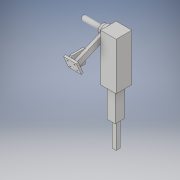
# Autodesk Inventor part: simp_burnisher
Saved by Autodesk Inventor 2019 (Build 230136000, 136)
## iProperties
Created: 2019-11-07
Part Number: simp_burnisher
Material: Generic
Document SubType Name: Modeling
Designer: luua
Density: 1 g/cm^3
Appearance: Default
Author: luua
Autodesk Inventor part; units mm, degrees
ref_plane "YZ Plane" through (0, 0, 0) normal (1, 0, 0) x (0, 1, 0)
ref_plane "XZ Plane" through (0, 0, 0) normal (0, 1, 0) x (-1, 0, 0)
ref_plane "XY Plane" through (0, 0, 0) normal (0, 0, 1) x (1, 0, 0)
sketch "Sketch1" plane through (0, 0, 0) normal (0, 0, 1) x (1, 0, 0)
  line L0 (-76.6085, 0) -> (76.6085, 0) construction
  line L1 (-48, 0) -> (48, 0)
  line L2 (48, 0) -> (48, 11)
  line L3 (48, 11) -> (-48, 11)
  line L4 (-48, 11) -> (-48, 0)
  point P0 (0, 0)
  point P1 (0, 0)
  point P2 (0, 11)
  dimension "d0" = 96
  dimension "d1" = 11
  constraints: 10 end point, 2 horizontal, 2 midpoint, 2 parallel, 1 coincident, 1 perpendicular, 1 point on line, 1 vertical alignment
  measures "d0" distance of L2.end L3.end
  measures "d1" distance of L1.end L2.end
revolve "Revolution1" add sketch "Sketch1" angle 360 about axis through (-76.6085, 0, 0) along (1, 0, 0)
sketch "Sketch2" plane through (48, 0, 0) normal (1, 0, 0) x (0, 0, -1)
  circle A0 centre (0, 0) radius 22.5
  dimension "d3" = 45
  constraints: 1 centre point, 1 coincident
  measures "d3" diameter of A0
extrude "Extrusion1" add sketch "Sketch2" along normal blind 30
sketch "Sketch3" plane through (0, 0, 0) normal (0, 0, 1) x (1, 0, 0)
  line L0 (78, -22.5) -> (78, 22.5) projected
  line L1 (78, 27.5) -> (78, -212.5)
  line L2 (48, 22.5) -> (78, 22.5) projected
  line L3 (48, -22.5) -> (78, -22.5) projected
  line L4 (78, 27.5) -> (158, 27.5)
  line L5 (158, 27.5) -> (158, -212.5)
  line L6 (78, -212.5) -> (98, -212.5)
  line L7 (158, -212.5) -> (138, -212.5)
  line L8 (118, 27.5) -> (118, -212.5) construction
  line L9 (98, -212.5) -> (98, -362.5)
  line L10 (98, -362.5) -> (138, -362.5)
  line L11 (138, -362.5) -> (138, -212.5)
  line L12 (108, -362.5) -> (128, -362.5)
  line L13 (128, -362.5) -> (128, -492.5)
  line L14 (128, -492.5) -> (108, -492.5)
  line L15 (108, -492.5) -> (108, -362.5)
  line L16 (138, -212.5) -> (98, -212.5)
  point P0 (0, 0)
  point P1 (118, -362.5)
  dimension "d6" = 5
  dimension "d7" = 190
  dimension "d8" = 80
  dimension "d9" = 40
  dimension "d10" = 150
  dimension "d36" = 20
  dimension "d37" = 130
  constraints: 28 end point, 6 horizontal, 3 midpoint, 3 perpendicular, 3 vertical, 2 collinear, 2 parallel, 1 horizontal alignment, 1 symmetric about line
  measures "d6" distance from line of L1.start L2
  measures "d7" distance from line of L1.end L3
  measures "d8" distance of L1.start L4.end
  measures "d9" distance of L6.end L7.end
  measures "d10" distance of L6.end L9.end
  measures "d36" distance of L13.end L14.end
  measures "d37" distance of L12.end L13.end
extrude "Extrusion2" add sketch "Sketch3" along normal mid plane 80 contours L0 L1 L4 L5 L7 L16 L6
sketch "Sketch4" plane through (78, -212.5, 40) normal (-1, 0, 0) x (0, 0, 1)
  circle A0 centre (-40, 212.5) radius 22.5 projected
  circle A1 centre (-40, 212.5) radius 27.5
  line L0 (-12.6869, 215.7005) -> (123.729, 157.7954)
  line L1 (123.729, 157.7954) -> (112.0071, 130.1803)
  line L2 (112.0071, 130.1803) -> (-26.0686, 188.7899)
  line L3 (0, 240) -> (0, 0) projected
  dimension "d13" = 55
  dimension "d14" = 150
  dimension "d15" = 90
  dimension "d16" = 30
  dimension "d17" = 67
  constraints: 6 end point, 2 point on circle, 1 centre point, 1 coincident, 1 perpendicular
  measures "d13" diameter of A1
  measures "d14" distance of L1.end L2.end
  measures "d15" angle of L1 L2
  measures "d16" distance of L0.end L1.end
  measures "d17" angle of L3 L2
extrude "Extrusion3" add sketch "Sketch4" along normal blind 15
extrude "Extrusion7" add sketch "Sketch3" along normal mid plane 50 contours L16 L11 L10 L9
extrude "Extrusion8" add sketch "Sketch3" along normal mid plane 20 contours L10 L13 L14 L15
sketch "Sketch5" plane through (63, -212.5, 40) normal (-1, 0, 0) x (0, 0, 1)
  line L0 (62.2205, 183.9042) -> (130.5668, 183.9042)
  line L1 (105.1693, 114.0714) -> (62.2205, 114.0714)
  line L2 (62.2205, 114.0714) -> (62.2205, 183.9042)
  line L3 (123.729, 157.7954) -> (-12.6869, 215.7005) projected
  circle A0 centre (-40, 212.5) radius 22.5 projected
  arc A1 (-12.6869, 215.7005) -> (-26.0686, 188.7899) centre (-40, 212.5) ccw projected
  line L4 (-26.0686, 188.7899) -> (112.0071, 130.1803) projected
  line L5 (112.0071, 130.1803) -> (123.729, 157.7954) projected
  line L6 (123.729, 157.7954) -> (-12.6869, 215.7005) projected
  line L7 (130.5668, 173.9042) -> (105.1693, 114.0714)
  line L8 (105.1693, 114.0714) -> (114.3743, 110.1641)
  line L9 (114.3743, 110.1641) -> (139.7719, 169.9969)
  line L10 (139.7719, 169.9969) -> (130.5668, 173.9042)
  line L11 (112.0071, 130.1803) -> (123.729, 157.7954) projected
  line L12 (130.5668, 183.9042) -> (130.5668, 173.9042)
  point P0 (117.868, 143.9878)
  dimension "d45" = 65
  dimension "d46" = 10
  dimension "d48" = 10
  constraints: 16 end point, 3 parallel, 3 point on line, 2 midpoint, 2 perpendicular, 1 collinear, 1 horizontal, 1 vertical
  measures "d45" distance of L8.end L9.end
  measures "d46" distance between parallel lines of L7 L9
  measures "d48" distance of L0.end L7.start
extrude "Extrusion4" add sketch "Sketch5" along normal blind 10 contours L3 L5 L4 L2 | L0 L12 L7 L3 | L4 L7 L1 L2
extrude "Extrusion5" add sketch "Sketch5" along normal mid plane 65 contours L7 L10 L9 L8 L5
sketch "Sketch8" plane through (30.5, -42.5031, 179.7719) normal (0, -0.3907311, 0.9205049) x (1, 0, 0)
  circle A0 centre (14.6708, -14.9131) radius 3.25
  circle A1 centre (14.6708, -50.2685) radius 3.25
  circle A2 centre (50.0262, -50.2685) radius 3.25
  circle A3 centre (50.0262, -14.9131) radius 3.25
  circle A4 centre (57.3485, -32.5908) radius 3
  circle A5 centre (32.3485, -32.5908) radius 30.5
  circle A6 centre (32.3485, -32.5908) radius 16.75
  line L0 (65, 0) -> (0, 0) projected
  line L1 (0, -65) -> (0, 0) projected
  line L2 (65, -65) -> (0, -65) projected
  line L3 (65, 0) -> (65, -65) projected
  line L4 (65, 0) -> (0, -65) construction
  line L5 (0, 0) -> (65, -65) construction
  point P0 (32.5, -32.5)
  constraints: 7 centre point, 4 end point, 1 midpoint
extrude "Extrusion9" cut sketch "Sketch8" against normal blind 10 contours A0 | A1 | A2 | A3
ref_plane "Work Plane3" through (30.5, -72.4195, 167.0731) normal (0, -0.9205049, -0.3907311) x (1, 0, 0)
ref_plane "Work Plane4" through (63, -212.5, 40) normal (-1, 0, 0) x (0, 0, 1)
body "Solid1"
